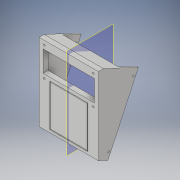
# Autodesk Inventor part: face
Saved by Autodesk Inventor 2017 (Build 210142000, 142)
## iProperties
Created: 2018-01-22
Part Number: face
Material: Generic
Document SubType Name: Modeling
Designer: chuck
Density: 1 g/cm^3
Appearance: Default
Author: chuck
Autodesk Inventor part; units mm, degrees
ref_plane "YZ Plane" through (0, 0, 0) normal (1, 0, 0) x (0, 1, 0)
ref_plane "XZ Plane" through (0, 0, 0) normal (0, 1, 0) x (-1, 0, 0)
ref_plane "XY Plane" through (0, 0, 0) normal (0, 0, 1) x (1, 0, 0)
sketch "Sketch1" plane through (0, 0, 0) normal (0, 0, 1) x (1, 0, 0)
  line L0 (0, 0) -> (112.522, 0)
  line L1 (112.522, 0) -> (112.522, 146.812)
  line L2 (112.522, 146.812) -> (0, 146.812)
  line L3 (0, 146.812) -> (0, 0)
  line L4 (7.62, 131.572) -> (104.902, 131.572)
  line L5 (104.902, 131.572) -> (104.902, 91.44)
  line L6 (104.902, 91.44) -> (7.62, 91.44)
  line L7 (7.62, 91.44) -> (7.62, 131.572)
  line L8 (21.59, 83.82) -> (90.932, 83.82)
  line L9 (90.932, 83.82) -> (90.932, 6.35)
  line L10 (90.932, 6.35) -> (21.59, 6.35)
  line L11 (21.59, 6.35) -> (21.59, 83.82)
  dimension "d0" = 97.282
  dimension "d1" = 40.132
  dimension "d2" = 69.342
  dimension "d3" = 77.47
  dimension "d4" = 6.35
  dimension "d5" = 21.59
  dimension "d6" = 7.62
  dimension "d7" = 7.62
  dimension "d8" = 15.24
  dimension "d9" = 7.62
  constraints: 24 end point, 6 parallel, 3 horizontal, 3 perpendicular
  measures "d0" distance of L4.start L4.end
  measures "d1" distance of L6.end L4.start
  measures "d2" distance of L8.start L8.end
  measures "d3" distance of L10.end L8.start
  measures "d4" distance between parallel lines of L0 L10
  measures "d5" distance between parallel lines of L3 L11
  measures "d6" distance between parallel lines of L3 L7
  measures "d7" distance between parallel lines of L1 L5
  measures "d8" distance between parallel lines of L2 L4
  measures "d9" distance between parallel lines of L6 L8
extrude "Extrusion1" add sketch "Sketch1" along normal blind 9.4996 contours L3 L2 L1 L0 | L8 L9 L10 L11
sketch "Sketch2" plane through (0, 0, 9.4996) normal (0, 0, 1) x (1, 0, 0)
  line L0 (0, 0) -> (112.522, 0)
  line L1 (112.522, 0) -> (112.522, 139.192)
  line L2 (112.522, 139.192) -> (0, 139.192)
  line L3 (0, 139.192) -> (0, 0)
  line L4 (7.62, 131.572) -> (104.902, 131.572)
  line L5 (104.902, 131.572) -> (104.902, 91.44)
  line L6 (104.902, 91.44) -> (7.62, 91.44)
  line L7 (7.62, 91.44) -> (7.62, 131.572)
  line L8 (21.59, 83.82) -> (90.932, 83.82)
  line L9 (90.932, 83.82) -> (90.932, 6.35)
  line L10 (90.932, 6.35) -> (21.59, 6.35)
  line L11 (21.59, 6.35) -> (21.59, 83.82)
  line L12 (20.32, 85.09) -> (92.202, 85.09)
  line L13 (92.202, 85.09) -> (92.202, 5.08)
  line L14 (92.202, 5.08) -> (20.32, 5.08)
  line L15 (20.32, 5.08) -> (20.32, 85.09)
  dimension "d12" = 97.282
  dimension "d13" = 40.132
  dimension "d14" = 69.342
  dimension "d15" = 77.47
  dimension "d16" = 6.35
  dimension "d17" = 21.59
  dimension "d18" = 7.62
  dimension "d19" = 7.62
  dimension "d20" = 7.62
  dimension "d21" = 7.62
  dimension "d33" = 1.27
  dimension "d34" = 1.27
  dimension "d35" = 1.27
  dimension "d36" = 1.27
  constraints: 32 end point, 8 parallel, 4 horizontal, 4 perpendicular
  measures "d12" distance of L4.start L4.end
  measures "d13" distance of L6.end L4.start
  measures "d14" distance of L8.start L8.end
  measures "d15" distance of L10.end L8.start
  measures "d16" distance between parallel lines of L0 L10
  measures "d17" distance between parallel lines of L3 L11
  measures "d18" distance between parallel lines of L3 L7
  measures "d19" distance between parallel lines of L1 L5
  measures "d20" distance between parallel lines of L2 L4
  measures "d21" distance between parallel lines of L6 L8
  measures "d33" distance between parallel lines of L13 L9
  measures "d34" distance between parallel lines of L12 L8
  measures "d35" distance between parallel lines of L15 L11
  measures "d36" distance between parallel lines of L10 L14
extrude "Extrusion2" cut sketch "Sketch2" against normal blind 1.27 contours L12 L13 L14 L15
sketch "Sketch3" plane through (0, 0, 9.4996) normal (0, 0, 1) x (1, 0, 0)
  circle A0 centre (9.7155, 138.9888) radius 1.651
  circle A1 centre (102.7811, 138.9888) radius 1.651
  circle A2 centre (102.7811, 84.0232) radius 1.651
  circle A3 centre (9.7155, 84.0232) radius 1.651
  line L0 (104.902, 131.572) -> (104.902, 91.44) projected
  line L1 (104.902, 91.44) -> (7.62, 91.44) projected
  line L2 (21.59, 6.35) -> (90.932, 6.35) projected
  line L3 (92.202, 5.08) -> (20.32, 5.08) projected
  line L4 (46.101, 6.35) -> (66.421, 6.35)
  line L5 (66.421, 6.35) -> (66.421, 5.08)
  line L6 (66.421, 5.08) -> (46.101, 5.08)
  line L7 (46.101, 5.08) -> (46.101, 6.35)
  line L8 (21.59, 83.82) -> (21.59, 6.35) projected
  line L9 (90.932, 6.35) -> (90.932, 83.82) projected
  point P0 (0, 0)
  dimension "d24" = 3.302
  dimension "d25" = 93.0656
  dimension "d26" = 93.0656
  dimension "d27" = 0
  dimension "d28" = 54.9656
  dimension "d29" = 2.1209
  dimension "d30" = 0
  dimension "d31" = 7.4168
  dimension "d32" = 0
  dimension "d37" = 20.32
  dimension "d38" = 24.511
  dimension "d39" = 24.511
  constraints: 8 end point, 4 centre point, 3 equal radius, 2 parallel, 2 point on line, 1 horizontal, 1 perpendicular
  measures "d24" diameter of A1
  measures "d25" distance of A1.centre A0.centre
  measures "d26" distance of A2.centre A3.centre
  measures "d27" vertical distance of A2.centre A3.centre
  measures "d28" distance of A0.centre A3.centre
  measures "d29" distance from line of L0 A1.centre
  measures "d30" vertical distance of A1.centre A0.centre
  measures "d31" distance from line of L1 A2.centre
  measures "d32" horizontal distance of A0.centre A3.centre
  measures "d37" distance between parallel lines of L5 L7
  measures "d38" distance between parallel lines of L8 L7
  measures "d39" distance between parallel lines of L9 L5
extrude "Extrusion3" cut sketch "Sketch3" against normal through all
sketch "Sketch4" plane through (0, 0, 0) normal (0, 0, -1) x (-1, 0, 0)
  line L0 (-118.574, 80.01) -> (11.603, 80.01)
  line L1 (11.603, 80.01) -> (11.603, -11.4067)
  line L2 (11.603, -11.4067) -> (-118.574, -11.4067)
  line L3 (-118.574, -11.4067) -> (-118.574, 80.01)
  line L4 (0, 0) -> (-112.522, 0) projected
  dimension "d42" = 80.01
  constraints: 8 end point, 2 parallel, 1 horizontal, 1 perpendicular
  measures "d42" distance between parallel lines of L0 L4
extrude "Extrusion4" cut sketch "Sketch4" against normal blind 4.4196
sketch "Sketch5" plane through (112.522, 0, 9.4996) normal (1, 0, 0) x (0, 0, -1)
  line L0 (9.4996, 146.812) -> (0, 146.812) projected
  line L1 (9.4996, 146.812) -> (75.9867, 115.8086)
  line L2 (5.08, 0) -> (0, 0) projected
  line L3 (18.0577, -8.4205) -> (0, 0)
  line L4 (0, 146.812) -> (0, 0) projected
  line L5 (0, 0) -> (0, 146.812)
  line L6 (0, 146.812) -> (9.4996, 146.812)
  line L7 (75.9867, 115.8086) -> (18.0577, -8.4205)
  line L8 (22.86, 146.812) -> (22.86, 73.406)
  line L9 (9.4996, 80.01) -> (9.4996, 146.812) projected
  point P0 (9.4996, 0)
  point P1 (22.86, 80.01)
  dimension "d45" = 25
  dimension "d47" = 22.86
  dimension "d48" = 33.02
  constraints: 12 end point, 2 perpendicular, 1 collinear, 1 parallel, 1 point on line, 1 vertical
  measures "d45" angle of L0 L1
  measures "d47" distance between parallel lines of L8 L4
  measures "d48" distance from line of point (22.86, 80.01) L7
extrude "Extrusion5" add sketch "Sketch5" against normal blind 3.81
ref_plane "Work Plane1" through (56.261, 0, 9.4996) normal (-1, 0, 0) x (0, 0, 1)
mirror "Mirror1" about plane through (56.261, 0, 9.4996) normal (-1, 0, 0) of "Extrusion5"
sketch "Sketch7" plane through (112.522, 0, 9.4996) normal (1, 0, 0) x (0, 0, -1)
  line L0 (18.0577, -8.4205) -> (0, 0) projected
  line L1 (0, 0) -> (18.0577, -8.4205)
  line L2 (18.0577, -8.4205) -> (19.6679, -4.9674)
  line L3 (75.9867, 115.8086) -> (18.0577, -8.4205) projected
  line L4 (0, 4.2039) -> (0, 0)
  line L5 (1.27, 6.35) -> (1.27, 83.82) projected
  line L6 (19.6679, -4.9674) -> (0, 4.2039)
  line L7 (9.4996, 146.812) -> (0, 146.812) projected
  line L8 (9.4996, 146.812) -> (9.4996, 142.6081)
  line L9 (9.4996, 146.812) -> (9.4996, 80.01) projected
  line L10 (9.4996, 142.6081) -> (39.8462, 128.4573)
  line L11 (39.8462, 128.4573) -> (41.4564, 131.9103)
  line L12 (9.4996, 146.812) -> (75.9867, 115.8086) projected
  line L13 (41.4564, 131.9103) -> (9.4996, 146.812)
  point P0 (9.4996, 0)
  dimension "d51" = 3.81
  dimension "d61" = 3.81
  dimension "d63" = 38.1
  constraints: 16 end point, 3 perpendicular, 3 point on line, 1 collinear, 1 parallel
  measures "d51" distance between parallel lines of L6 L0
  measures "d61" distance between parallel lines of L12 L10
  measures "d63" distance from line of L3.start L11
extrude "Extrusion6" add sketch "Sketch7" against normal through all
sketch "Sketch8" plane through (112.522, 0, 9.4996) normal (1, 0, 0) x (0, 0, -1)
  circle A0 centre (19.1087, 5.1024) radius 1.5875
  circle A1 centre (66.3031, 106.3112) radius 1.5875
  line L0 (0, 0) -> (18.0577, -8.4205) projected
  line L1 (18.0577, -8.4205) -> (75.9867, 115.8086) projected
  line L2 (75.9867, 115.8086) -> (9.4996, 146.812) projected
  point P0 (9.4996, 0)
  dimension "d54" = 3.175
  dimension "d55" = 12.7
  dimension "d56" = 4.7625
  dimension "d57" = 4.7625
  dimension "d58" = 12.7
  constraints: 2 centre point, 1 equal radius
  measures "d54" diameter of A0
  measures "d55" distance from line of A0.centre L0
  measures "d56" distance from line of A0.centre L1
  measures "d57" distance from line of L1 A1.centre
  measures "d58" distance from line of L2 A1.centre
extrude "Extrusion7" cut sketch "Sketch8" against normal through all
body "Solid1"
